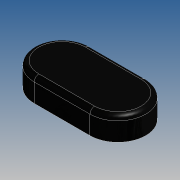
# Autodesk Inventor part: F113PrisePile
Saved by Autodesk Inventor 2015 SP1 (Build 190203100, 203)
## iProperties
Created: 2017-01-26
Part Number: F113PrisePile
Material: ABS Plastic
Document SubType Name: Modeling
Designer: serge.amoos
Density: 1.06 g/cm^3
Appearance: Smooth - Black
Author: serge.amoos
Autodesk Inventor part; units mm, degrees
ref_plane "YZ Plane" through (0, 0, 0) normal (1, 0, 0) x (0, 1, 0)
ref_plane "XZ Plane" through (0, 0, 0) normal (0, 1, 0) x (-1, 0, 0)
ref_plane "XY Plane" through (0, 0, 0) normal (0, 0, 1) x (1, 0, 0)
sketch "Sketch1" plane through (0, 0, 0) normal (0, 0, 1) x (1, 0, 0)
  line L0 (-14.4, 0) -> (2.4, 0) projected
  line L1 (0, -8.4) -> (0, 8.4) projected
  line L2 (0, 6) -> (-6, 6)
  line L3 (-6, 6) -> (-6, -6)
  line L4 (-6, -6) -> (0, -6)
  line L5 (0, -6) -> (0, 6)
  arc A0 (-6, 6) -> (-6, -6) centre (-6, 0) ccw
  point P0 (0, 0)
  dimension "d0" = 12
  dimension "d1" = 6
  constraints: 8 end point, 2 midpoint, 2 parallel, 2 point on circle, 1 centre point, 1 coincident, 1 horizontal, 1 perpendicular, 1 point on line
  measures "d0" distance of L2.end L3.end
  measures "d1" distance of L2.start L2.end
extrude "Extrusion1" add sketch "Sketch1" along normal blind 5
fillet "Fillet1" radius 1 3 edges at (-3, -6, 5) (-3, 6, 5) (-12, 0, 5)
mirror "Mirror1" about plane through (0, -6, 0) normal (1, 0, 0)
body "Solid1"
